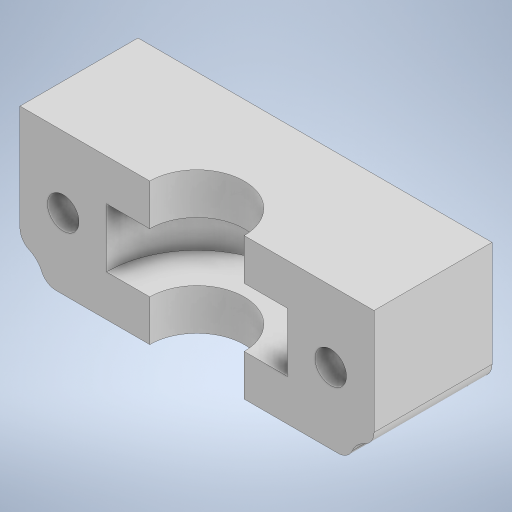
# Autodesk Inventor part: bearing_holder_top_test_v1
Saved by Autodesk Inventor 2024 (Build 280153000, 153)
## iProperties
Created: 2024-02-02
Part Number: bearing_holder_top_test_v1
Material: Generic
Document SubType Name: Modeling
Designer: Pintu
Density: 1 g/cm^3
Appearance: Default
Mass: 12.15 g
Surface Area: 35.1 cm^2
Volume: 12.15 cm^3
Author: Pintu
Autodesk Inventor part; units mm, degrees
ref_plane "YZ Plane" through (0, 0, 0) normal (1, 0, 0) x (0, 1, 0)
ref_plane "XZ Plane" through (0, 0, 0) normal (0, 1, 0) x (-1, 0, 0)
sketch "Sketch1" plane through (0, 0, 0) normal (0, 0, 1) x (1, 0, 0)
  line L0 (-22.5, 9) -> (22.5, 9)
  line L1 (22.5, 9) -> (22.5, -9)
  line L2 (22.5, -9) -> (-22.5, -9)
  line L3 (-22.5, -9) -> (-22.5, 9)
  line L4 (-22.5, 9) -> (22.5, -9) construction
  line L5 (22.5, 9) -> (-22.5, -9) construction
  point P0 (0, 0)
  dimension "d0" = 45
  dimension "d1" = 18
  constraints: 12 end point, 2 midpoint, 2 parallel, 1 horizontal, 1 perpendicular
  measures "d0" distance of L1.end L2.end
  measures "d1" distance of L0.end L1.end
extrude "Extrusion1" add sketch "Sketch1" along normal blind 15
ref_plane "Work Plane2" through (-22.5, 0, 0) normal (0, -1, 0) x (1, 0, 0)
sketch "Sketch4" plane through (-22.5, 0, 0) normal (0, -1, 0) x (1, 0, 0)
  line L0 (0, 15) -> (45, 15) projected
  circle A0 centre (22.5, 15) radius 11.5
  point P0 (22.5, 0)
  dimension "d6" = 23
  constraints: 1 centre point, 1 midpoint
  measures "d6" diameter of A0
extrude "Extrusion2" cut sketch "Sketch4" along normal mid plane 7.5
sketch "Sketch5" plane through (-22.5, 0, 0) normal (0, -1, 0) x (1, 0, 0)
  line L0 (45, 0) -> (0, 0) projected
  line L1 (0, 0) -> (0, 15) projected
  line L2 (45, 15) -> (0, 15) projected
  line L3 (45, 0) -> (45, 15) projected
  line L4 (11, 15) -> (34, 15) projected
  arc A0 (11, 15) -> (34, 15) centre (22.5, 15) ccw projected
  circle A1 centre (22.5, 15) radius 6
  point P0 (22.5, 0)
  dimension "d9" = 12
  constraints: 1 centre point, 1 coincident
  measures "d9" diameter of A1
extrude "Extrusion3" cut sketch "Sketch5" along normal mid plane 31.5 contours A1 L2 | L2 A1
fillet "Fillet1" radius 3 2 edges at (-22.5, -9, 7.5) (22.5, -9, 7.5) inverted yes
fillet "Fillet2" radius 2 4 edges at (-19.5, -9, 7.5) (-22.5, -6, 7.5) (19.5, -9, 7.5) (22.5, -6, 7.5)
sketch "Sketch8" plane through (0, 0, 0) normal (0, 0, -1) x (-1, 0, 0)
  line L0 (22.5, 9) -> (22.5, -4.4174) projected
  line L1 (17.9174, -9) -> (-17.9174, -9) projected
  point P0 (0, 0)
  point P1 (17, 0)
  dimension "sideOff" = 5.5
  dimension "d33" = 9
  measures "sideOff" distance from line of L0 point (17, 0)
  measures "d33" distance from line of L1 point (17, 0)
hole "Hole3" at (-17, 0, 0) direction (0, 0, 1) diameter 4 depth 25 tip angle 118
sketch "Sketch9" plane through (0, 0, 0) normal (0, 0, -1) x (-1, 0, 0)
  line L0 (-22.5, -4.4174) -> (-22.5, 9) projected
  line L1 (17.9174, -9) -> (-17.9174, -9) projected
  point P0 (0, 0)
  point P1 (-17, 0)
  dimension "d41" = 5.5
  dimension "d42" = 9
  measures "d41" distance from line of L0 point (-17, 0)
  measures "d42" distance from line of L1 point (-17, 0)
hole "Hole4" at (17, 0, 0) direction (0, 0, 1) diameter 4 depth 25 tip angle 118
sketch "Sketch10" plane through (0, 0, 0) normal (0, 0, -1) x (-1, 0, 0)
  circle A0 centre (17, 0) radius 2 projected
  circle A1 centre (-17, 0) radius 2 projected
  line L0 (14.8349, 3.75) -> (19.1651, 3.75)
  line L1 (19.1651, 3.75) -> (21.3301, 0)
  line L2 (21.3301, 0) -> (19.1651, -3.75)
  line L3 (19.1651, -3.75) -> (14.8349, -3.75)
  line L4 (14.8349, -3.75) -> (12.6699, 0)
  line L5 (12.6699, 0) -> (14.8349, 3.75)
  line L6 (-19.1651, 3.75) -> (-14.8349, 3.75)
  line L7 (-14.8349, 3.75) -> (-12.6699, 0)
  line L8 (-12.6699, 0) -> (-14.8349, -3.75)
  line L9 (-14.8349, -3.75) -> (-19.1651, -3.75)
  line L10 (-19.1651, -3.75) -> (-21.3301, 0)
  line L11 (-21.3301, 0) -> (-19.1651, 3.75)
  line L12 (-22.5, 9) -> (22.5, 9) projected
  point P0 (0, 0)
  point P1 (17, -3.75)
  point P2 (17, 3.75)
  point P3 (-17, 3.75)
  point P4 (-17, -3.75)
  dimension "nut" = 7.5
  dimension "d51" = 7.5
  constraints: 24 end point, 4 midpoint, 2 coincident, 2 parallel, 26 other
  measures "nut" distance of point (17, -3.75) point (17, 3.75)
  measures "d51" distance of point (-17, 3.75) point (-17, -3.75)
extrude "Extrusion4" cut sketch "Sketch10" against normal blind 8
equation "\"d41\" = sideOff"
equation "\"d51\" = nut"
body "Solid1"
